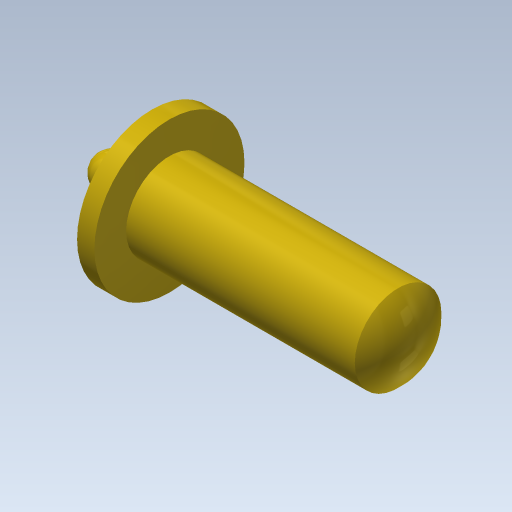
# Autodesk Inventor part: Pump-Motor-CW-Rotation:Follower
Saved by Autodesk Inventor 2024.2 (Build 282272000, 272)
## iProperties
Created: 2025-06-16
Document SubType Name: Modeling
Density: 7.73 g/cm^3
Material: Steel, Alloy
Mass: 70.8626 g
Surface Area: 33.6984 cm^2
Volume: 9.16721 cm^3
Appearance: Glossy - Gold
Designer: cw
Author: cw
Autodesk Inventor part; units mm, degrees
ref_plane "YZ Plane" through (0, 0, 0) normal (1, 0, 0) x (0, 1, 0)
ref_plane "XZ Plane" through (0, 0, 0) normal (0, 1, 0) x (-1, 0, 0)
ref_plane "XY Plane" through (0, 0, 0) normal (0, 0, 1) x (1, 0, 0)
sketch "Sketch1" plane through (0, 0, 0) normal (0, 0, 1) x (1, 0, 0)
  arc A0 (10, 0) -> (6.6144, 7.5) centre (0, 0) ccw
  line L0 (6.6144, 7.5) -> (-33, 7.5)
  line L1 (-33, 7.5) -> (-33, 13)
  line L2 (-33, 13) -> (-36, 13)
  line L3 (-36, 13) -> (-36, 3)
  line L4 (-36, 3) -> (-43, 3)
  arc A1 (-43, 3) -> (-46, 0) centre (-43, 0) ccw
  line L5 (10, 0) -> (-46, 0)
  dimension "d1" = 13
  dimension "d2" = 3
  dimension "d3" = 3
  dimension "d7" = 10
  dimension "d9" = 7.5
  dimension "d10" = 43
  dimension "d11" = 10
  dimension "d13" = 3.3856
  constraints: 12 end point, 4 parallel, 4 point on circle, 2 centre point, 2 point on line, 1 coincident, 1 horizontal, 1 perpendicular, 1 tangent
  measures "d1" distance between parallel lines of L5 L2
  measures "d2" radius of A1
  measures "d3" distance of L1.end L2.end
  measures "d7" distance from line of L5.end L3
  measures "d9" distance between parallel lines of L5 L0
  measures "d10" distance from line of L5.start L1
  measures "d11" radius of A0
  measures "d13" horizontal distance of L0.start L5.start
revolve "Revolution1" add sketch "Sketch1" angle 360 about axis through (10, 0, 0) along (-1, 0, 0)
body "Solid1"
